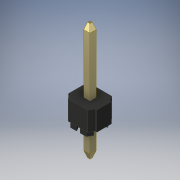
# Autodesk Inventor part: C-Pin
Saved by Autodesk Inventor 2017 (Build 210142000, 142)
## iProperties
Created: 2016-07-07
Part Number: C-Pin
Material: Generic
Document SubType Name: Modeling
Designer: Home
Density: 1 g/cm^3
Appearance: Default
Author: Home
Autodesk Inventor part; units mm, degrees
ref_plane "YZ Plane" through (0, 0, 0) normal (1, 0, 0) x (0, 1, 0)
ref_plane "XZ Plane" through (0, 0, 0) normal (0, 1, 0) x (-1, 0, 0)
ref_plane "XY Plane" through (0, 0, 0) normal (0, 0, 1) x (1, 0, 0)
sketch "Sketch1" plane through (0, 0, 0) normal (0, 1, 0) x (-1, 0, 0)
  line L0 (1.02, 1.25) -> (1.27, 0.75)
  line L1 (-1.02, 1.25) -> (1.02, 1.25)
  line L2 (-1.27, -0.75) -> (-1.27, 0.75)
  line L3 (-1.02, -1.25) -> (-1.27, -0.75)
  line L4 (1.02, -1.25) -> (-1.02, -1.25)
  line L5 (1.27, -0.75) -> (1.02, -1.25)
  line L6 (1.27, 0.75) -> (1.27, -0.75)
  line L7 (1.02, 1.25) -> (1.27, 0.75)
  line L8 (-1.02, 1.25) -> (1.02, 1.25)
  line L9 (-1.27, 0.75) -> (-1.02, 1.25)
  line L10 (0.815, 1.2) -> (0.18, 1.2)
  line L11 (1.1037, 0.7) -> (0.815, 1.2)
  line L12 (0.4687, 0.7) -> (1.1037, 0.7)
  line L13 (0.18, 1.2) -> (0.4687, 0.7)
  line L14 (-0.815, 1.2) -> (-1.1037, 0.7)
  line L15 (-0.18, 1.2) -> (-0.815, 1.2)
  line L16 (-0.4687, 0.7) -> (-0.18, 1.2)
  line L17 (-1.1037, 0.7) -> (-0.4687, 0.7)
  line L18 (0.815, -1.2) -> (1.1037, -0.7)
  line L19 (0.18, -1.2) -> (0.815, -1.2)
  line L20 (0.4687, -0.7) -> (0.18, -1.2)
  line L21 (1.1037, -0.7) -> (0.4687, -0.7)
  line L22 (-0.815, -1.2) -> (-0.18, -1.2)
  line L23 (-1.1037, -0.7) -> (-0.815, -1.2)
  line L24 (-0.4687, -0.7) -> (-1.1037, -0.7)
  line L25 (-0.18, -1.2) -> (-0.4687, -0.7)
  line L26 (-0.325, 0.325) -> (0.325, 0.325)
  line L27 (0.325, 0.325) -> (0.325, -0.325)
  line L28 (-0.325, -0.325) -> (0.325, -0.325)
  line L29 (-0.325, 0.325) -> (-0.325, -0.325)
  point P0 (0, 0)
  point P1 (0, 0)
  constraints: 60 end point, 18 parallel, 1 horizontal, 1 vertical
sketch "Sketch3" plane through (0, 0, 0) normal (0, 1, 0) x (-1, 0, 0)
  line L0 (1.1062, -0.7) -> (0.4712, -0.7)
  line L1 (0.4712, -0.7) -> (0.1825, -1.2)
  line L2 (0.1825, -1.2) -> (0.8175, -1.2)
  line L3 (0.8175, -1.2) -> (1.1062, -0.7)
  line L4 (0.5, -1.2) -> (0.5, -0.7) construction
  point P0 (0, 0)
  dimension "d58" = 120
  dimension "d60" = 0.7
  dimension "d61" = 0.635
  dimension "d62" = 0.5
  dimension "d65" = 0.5
  constraints: 10 end point, 2 parallel, 1 horizontal, 1 midpoint, 1 perpendicular, 1 point on line
  measures "d58" angle of L1 L0
  measures "d60" distance from line of L0 point (0, 0)
  measures "d61" distance of L1.end L2.end
  measures "d62" vertical distance of L2.end L0.start
  measures "d65" distance from line of point (0, 0) L4
extrude "PCB-Level" add sketch "Sketch3" along normal blind 0.5
mirror "PCB-Level-Mirror1" about plane through (0, 0, 0) normal (1, 0, 0) of "PCB-Level"
mirror "PCB_Level-Mirror2" about plane through (0, 0, 0) normal (0, 0, 1) of "PCB-Level", "PCB-Level-Mirror1"
sketch "Sketch4" plane through (0, 0.5, 0) normal (0, 1, 0) x (1, 0, 0)
  line L0 (-1.02, -1.25) -> (1.02, -1.25)
  line L1 (1.27, -0.75) -> (1.27, 0.75)
  line L2 (1.02, 1.25) -> (-1.02, 1.25)
  line L3 (-1.27, 0.75) -> (-1.27, -0.75)
  line L4 (-1.27, -1.25) -> (1.27, 1.25) construction
  line L5 (1.27, -1.25) -> (-1.27, 1.25) construction
  line L6 (1.27, -0.75) -> (1.02, -1.25)
  line L7 (1.27, 0.75) -> (1.02, 1.25)
  line L8 (-1.27, 0.75) -> (-1.02, 1.25)
  line L9 (-1.27, -0.75) -> (-1.02, -1.25)
  line L10 (-1.02, -1.25) -> (1.02, -1.25)
  line L11 (1.27, 0.75) -> (1.47, 0.75)
  line L12 (1.47, 0.75) -> (1.47, -0.75)
  line L13 (1.47, -0.75) -> (1.27, -0.75)
  line L14 (1.27, -0.75) -> (1.27, 0.75)
  line L15 (-1.27, -0.75) -> (-1.47, -0.75)
  line L16 (-1.47, -0.75) -> (-1.47, 0.75)
  line L17 (-1.47, 0.75) -> (-1.27, 0.75)
  line L18 (-1.27, 0.75) -> (-1.27, -0.75)
  point P0 (0, 0)
  dimension "d68" = 2.54
  dimension "d69" = 2.5
  dimension "d70" = 0.5
  dimension "d71" = 0.25
  dimension "d72" = 0.5
  dimension "d73" = 0.25
  dimension "d74" = 0.5
  dimension "d75" = 0.25
  dimension "d76" = 0.5
  dimension "d77" = 0.25
  dimension "d122" = 0.2
  dimension "d123" = 0.2
  constraints: 38 end point, 8 point on line, 6 parallel, 4 horizontal, 3 perpendicular, 2 midpoint
  measures "d68" distance of L5.end L4.end
  measures "d69" distance of L4.end L5.start
  measures "d70" distance of L1.start L5.start
  measures "d71" distance of L0.end L5.start
  measures "d72" distance of L1.end L4.end
  measures "d73" distance of L2.start L4.end
  measures "d74" distance of L3.start L5.end
  measures "d75" distance of L2.end L5.end
  measures "d76" distance of L3.end L4.start
  measures "d77" distance of L0.start L4.start
  measures "d122" distance of L12.end L13.end
  measures "d123" distance of L16.end L17.end
sketch "Sketch6" plane through (0, 0, 0) normal (0, 1, 0) x (-1, 0, 0)
  line L0 (0.325, -0.325) -> (-0.325, -0.325) projected
  line L1 (-0.325, -0.325) -> (-0.325, 0.325) projected
  line L2 (-0.325, 0.325) -> (0.325, 0.325) projected
  line L3 (0.325, 0.325) -> (0.325, -0.325) projected
  point P0 (0, 0)
extrude "Pin-Ext" add sketch "Sketch6" along normal blind 9.25 and the other way blind 2.9 separate body
chamfer "Chamfer1" distance 0.2 distance2 0.65 1 edges at (0, 9.25, -0.325) measured on face at (-0.1083, 9.25, -0.1083)
chamfer "Chamfer2" distance 0.2 distance2 0.65 1 edges at (-0.325, 9.25, 0.1) measured on face at (0.1083, 9.25, 0.175)
chamfer "Chamfer3" distance 0.2 distance2 0.65 1 edges at (0.1, 9.25, 0.325) measured on face at (0.175, 9.25, 0.175)
chamfer "Chamfer4" distance 0.2 distance2 0.65 1 edges at (0.325, 9.25, 0) measured on face at (0.175, 9.25, 0.0417)
chamfer "Chamfer5" distance 0.2 distance2 0.65 1 edges at (-0.325, -2.9, 0) measured on face at (-0.1083, -2.9, -0.1083)
chamfer "Chamfer6" distance 0.2 distance2 0.65 1 edges at (0.1, -2.9, 0.325) measured on face at (0.025, -2.9, -0.1083)
chamfer "Chamfer7" distance 0.2 distance2 0.65 1 edges at (0.1, -2.9, -0.325) measured on face at (0.025, -2.9, -0.175)
chamfer "Chamfer8" distance 0.2 distance2 0.65 1 edges at (0.325, -2.9, 0) measured on face at (0.025, -2.9, -0.0417)
extrude "Extrusion9" add sketch "Sketch4" along normal blind 2 bodies 1
sketch "Sketch9" plane through (0, 2.5, 0) normal (0, 1, 0) x (1, 0, 0)
  line L0 (0.325, 0.325) -> (-0.325, 0.325) projected
  line L1 (0.325, -0.325) -> (0.325, 0.325) projected
  line L2 (-0.325, -0.325) -> (0.325, -0.325) projected
  line L3 (-0.325, 0.325) -> (-0.325, -0.325) projected
  point P0 (0, 0)
extrude "Extrusion10" cut sketch "Sketch9" against normal through all bodies 1
equation "\"d74\" = d72"
equation "\"d75\" = d73"
equation "\"d76\" = d72"
equation "\"d77\" = d73"
